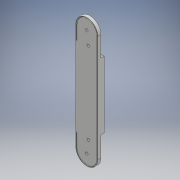
# Autodesk Inventor part: C-PAN-TOP
Saved by Autodesk Inventor 2018 (Build 220112000, 112)
## iProperties
Created: 2018-01-23
Part Number: C-PAN-TOP
Material: Generic
Document SubType Name: Modeling
Designer: gevon
Density: 1 g/cm^3
Appearance: Default
Author: gevon
Autodesk Inventor part; units mm, degrees
ref_plane "YZ Plane" through (0, 0, 0) normal (1, 0, 0) x (0, 1, 0)
ref_plane "XZ Plane" through (0, 0, 0) normal (0, 1, 0) x (-1, 0, 0)
ref_plane "XY Plane" through (0, 0, 0) normal (0, 0, 1) x (1, 0, 0)
sketch "Sketch1" plane through (0, 0, 0) normal (0, 1, 0) x (-1, 0, 0)
  arc A0 (17.5, 106.9997) -> (-17.5, 106.9997) centre (0, 106.9997) ccw
  arc A1 (-17.5, -63.0003) -> (17.5, -63.0003) centre (0, -63.0003) ccw
  line L0 (17.5, 106.9997) -> (17.5, -63.0003)
  line L1 (-17.5, 106.9997) -> (-17.5, -63.0003)
  circle A2 centre (0, 106.9997) radius 2
  circle A3 centre (0, -63.0003) radius 2
  point P0 (0, 0)
  dimension "d0" = 35
  dimension "d1" = 35
  dimension "d2" = 205
  dimension "d3" = 4
  dimension "d4" = 4
  constraints: 4 centre point, 4 end point, 4 point on circle, 2 coincident, 2 tangent, 2 vertical
  measures "d0" diameter of A0
  measures "d1" diameter of A1
  measures "d3" diameter of A2
  measures "d4" diameter of A3
extrude "Extrusion1" add sketch "Sketch1" along normal blind 5
sketch "Sketch2" plane through (0, 5, 0) normal (0, 1, 0) x (1, 0, 0)
  circle A0 centre (2.5, 43.0003) radius 2
  circle A1 centre (2.5, -86.9997) radius 2
  line L0 (-17.5, 63.0003) -> (-17.5, -106.9997) projected
  circle A2 centre (0, 63.0003) radius 2 projected
  circle A3 centre (0, -106.9997) radius 2 projected
  point P0 (0, 0)
  dimension "d7" = 4
  dimension "d8" = 4
  dimension "d9" = 20
  dimension "d10" = 20
  dimension "d11" = 20
  constraints: 2 centre point
  measures "d7" diameter of A0
  measures "d8" diameter of A1
  measures "d9" distance from line of L0 A0.centre
  measures "d10" vertical distance of A2.centre A0.centre
  measures "d11" vertical distance of A3.centre A1.centre
extrude "Extrusion2" cut sketch "Sketch2" against normal blind 5 contours A0 | A1
sketch "Sketch3" plane through (0, 5, 0) normal (0, 1, 0) x (1, 0, 0)
  line L0 (-17.5, 63.0003) -> (-17.5, -106.9997) projected
  line L1 (17.5, -106.9997) -> (17.5, 63.0003) projected
  line L2 (-17.5, 31.0003) -> (17.5, 31.0003)
  line L3 (17.5, 31.0003) -> (17.5, -74.9997)
  line L4 (17.5, -74.9997) -> (-17.5, -74.9997)
  line L5 (-17.5, -74.9997) -> (-17.5, 31.0003)
  circle A0 centre (2.5, 43.0003) radius 2 projected
  circle A1 centre (2.5, -86.9997) radius 2 projected
  point P0 (0, 0)
  dimension "d14" = 12
  dimension "d15" = 12
  constraints: 8 end point, 2 parallel, 2 point on line, 1 horizontal, 1 perpendicular
  measures "d14" distance from line of L2 A0.centre
  measures "d15" distance from line of L4 A1.centre
extrude "Extrusion3" add sketch "Sketch3" along normal blind 5 contours L2 L1 L4 L0
sketch "Sketch4" plane through (0, 10, 0) normal (0, 1, 0) x (1, 0, 0)
  point P0 (0, 0)
sketch "Sketch5" plane through (0, 10, 0) normal (0, 1, 0) x (1, 0, 0)
  line L0 (-10.4855, -70.1364) -> (34.9467, -70.1364) construction
  line L1 (34.9467, -70.1364) -> (34.9467, -84.8837) construction
  line L2 (34.9467, -84.8837) -> (-10.4855, -84.8837) construction
  line L3 (-10.4855, -84.8837) -> (-10.4855, -70.1364) construction
  spline S0 degree 2 poles (-8.9862, -73.3005) (-9.2826, -73.3005) (-9.784, -73.1004) (-9.9668, -72.9004) knots 0 0 0 1 2 2 2
  spline S1 degree 2 poles (-9.9668, -72.9004) (-10.1495, -72.7028) (-10.3496, -72.1099) (-10.3496, -71.7246) knots 0 0 0 1 2 2 2
  spline S2 degree 2 poles (-10.3496, -71.7246) (-10.3496, -71.3418) (-10.1545, -70.7737) (-9.9692, -70.5637) knots 0 0 0 1 2 2 2
  spline S3 degree 2 poles (-9.9692, -70.5637) (-9.7864, -70.3587) (-9.2875, -70.1438) (-8.9788, -70.1438) knots 0 0 0 1 2 2 2
  spline S4 degree 2 poles (-8.9788, -70.1438) (-8.8256, -70.1438) (-8.5564, -70.1883) (-8.4428, -70.2229) knots 0 0 0 1 2 2 2
  spline S5 degree 2 poles (-8.4428, -70.2229) (-8.344, -70.255) (-8.1389, -70.3464) (-8.0377, -70.4007) knots 0 0 0 1 2 2 2
  line L4 (-8.0377, -70.4007) -> (-8.0377, -70.8898)
  line L5 (-8.0377, -70.8898) -> (-8.0698, -70.8898)
  spline S6 degree 2 poles (-8.0698, -70.8898) (-8.1241, -70.8404) (-8.2921, -70.702) (-8.4131, -70.6353) knots 0 0 0 1 2 2 2
  spline S7 degree 2 poles (-8.4131, -70.6353) (-8.5292, -70.5711) (-8.8034, -70.4896) (-8.9812, -70.4896) knots 0 0 0 1 2 2 2
  spline S8 degree 2 poles (-8.9812, -70.4896) (-9.1764, -70.4896) (-9.5246, -70.6502) (-9.6555, -70.8033) knots 0 0 0 1 2 2 2
  spline S9 degree 2 poles (-9.6555, -70.8033) (-9.784, -70.9589) (-9.9272, -71.4307) (-9.9272, -71.7246) knots 0 0 0 1 2 2 2
  spline S10 degree 2 poles (-9.9272, -71.7246) (-9.9272, -72.0383) (-9.7766, -72.4903) (-9.6457, -72.6459) knots 0 0 0 1 2 2 2
  spline S11 degree 2 poles (-9.6457, -72.6459) (-9.5172, -72.7966) (-9.1739, -72.9498) (-8.9812, -72.9498) knots 0 0 0 1 2 2 2
  spline S12 degree 2 poles (-8.9812, -72.9498) (-8.8059, -72.9498) (-8.507, -72.8633) (-8.3909, -72.7991) knots 0 0 0 1 2 2 2
  spline S13 degree 2 poles (-8.3909, -72.7991) (-8.2797, -72.7349) (-8.1142, -72.6015) (-8.0673, -72.5546) knots 0 0 0 1 2 2 2
  line L6 (-8.0673, -72.5546) -> (-8.0377, -72.5546)
  line L7 (-8.0377, -72.5546) -> (-8.0377, -73.0387)
  spline S14 degree 2 poles (-8.0377, -73.0387) (-8.1389, -73.0856) (-8.3168, -73.1721) (-8.4428, -73.2116) knots 0 0 0 1 2 2 2
  spline S15 degree 2 poles (-8.4428, -73.2116) (-8.5761, -73.256) (-8.8034, -73.3005) (-8.9862, -73.3005) knots 0 0 0 1 2 2 2
  line L8 (-6.6298, -72.0976) -> (-7.7833, -72.0976)
  line L9 (-7.7833, -72.0976) -> (-7.7833, -71.7271)
  line L10 (-7.7833, -71.7271) -> (-6.6298, -71.7271)
  line L11 (-6.6298, -71.7271) -> (-6.6298, -72.0976)
  spline S16 degree 2 poles (-4.2116, -71.117) (-4.2116, -71.3146) (-4.3524, -71.6703) (-4.4784, -71.7938) knots 0 0 0 1 2 2 2
  spline S17 degree 2 poles (-4.4784, -71.7938) (-4.6365, -71.9494) (-5.0638, -72.1099) (-5.3898, -72.1099) knots 0 0 0 1 2 2 2
  line L12 (-5.3898, -72.1099) -> (-5.7332, -72.1099)
  line L13 (-5.7332, -72.1099) -> (-5.7332, -73.2462)
  line L14 (-5.7332, -73.2462) -> (-6.1382, -73.2462)
  line L15 (-6.1382, -73.2462) -> (-6.1382, -70.1982)
  line L16 (-6.1382, -70.1982) -> (-5.3725, -70.1982)
  spline S18 degree 2 poles (-5.3725, -70.1982) (-5.1008, -70.1982) (-4.7204, -70.2871) (-4.5747, -70.3883) knots 0 0 0 1 2 2 2
  spline S19 degree 2 poles (-4.5747, -70.3883) (-4.4043, -70.5044) (-4.2116, -70.8626) (-4.2116, -71.117) knots 0 0 0 1 2 2 2
  spline S20 degree 2 poles (-4.634, -71.1294) (-4.634, -70.9713) (-4.7427, -70.7391) (-4.8538, -70.665) knots 0 0 0 1 2 2 2
  spline S21 degree 2 poles (-4.8538, -70.665) (-4.9502, -70.6008) (-5.207, -70.5489) (-5.3972, -70.5489) knots 0 0 0 1 2 2 2
  line L17 (-5.3972, -70.5489) -> (-5.7332, -70.5489)
  line L18 (-5.7332, -70.5489) -> (-5.7332, -71.7641)
  line L19 (-5.7332, -71.7641) -> (-5.4565, -71.7641)
  spline S22 degree 2 poles (-5.4565, -71.7641) (-5.2095, -71.7641) (-4.9057, -71.6851) (-4.8069, -71.5814) knots 0 0 0 1 2 2 2
  spline S23 degree 2 poles (-4.8069, -71.5814) (-4.7155, -71.49) (-4.634, -71.2751) (-4.634, -71.1294) knots 0 0 0 1 2 2 2
  line L20 (-4.1548, -73.2462) -> (-3.1273, -70.1982)
  line L21 (-3.1273, -70.1982) -> (-2.6283, -70.1982)
  line L22 (-2.6283, -70.1982) -> (-1.6008, -73.2462)
  line L23 (-1.6008, -73.2462) -> (-2.0281, -73.2462)
  line L24 (-2.0281, -73.2462) -> (-2.3048, -72.394)
  line L25 (-2.3048, -72.394) -> (-3.4681, -72.394)
  line L26 (-3.4681, -72.394) -> (-3.7448, -73.2462)
  line L27 (-3.7448, -73.2462) -> (-4.1548, -73.2462)
  line L28 (-2.4159, -72.0482) -> (-2.8877, -70.6131)
  line L29 (-2.8877, -70.6131) -> (-3.357, -72.0482)
  line L30 (-3.357, -72.0482) -> (-2.4159, -72.0482)
  line L31 (0.8692, -73.2462) -> (0.4147, -73.2462)
  line L32 (0.4147, -73.2462) -> (-0.9339, -70.6181)
  line L33 (-0.9339, -70.6181) -> (-0.9339, -73.2462)
  line L34 (-0.9339, -73.2462) -> (-1.3118, -73.2462)
  line L35 (-1.3118, -73.2462) -> (-1.3118, -70.1982)
  line L36 (-1.3118, -70.1982) -> (-0.7363, -70.1982)
  line L37 (-0.7363, -70.1982) -> (0.4913, -72.6114)
  line L38 (0.4913, -72.6114) -> (0.4913, -70.1982)
  line L39 (0.4913, -70.1982) -> (0.8692, -70.1982)
  line L40 (0.8692, -70.1982) -> (0.8692, -73.2462)
  line L41 (4.4359, -73.2462) -> (2.949, -73.2462)
  line L42 (2.949, -73.2462) -> (2.949, -72.9349)
  line L43 (2.949, -72.9349) -> (3.5022, -72.9349)
  line L44 (3.5022, -72.9349) -> (3.5022, -70.8922)
  line L45 (3.5022, -70.8922) -> (2.949, -70.8922)
  line L46 (2.949, -70.8922) -> (2.949, -70.6131)
  spline S24 degree 2 poles (2.949, -70.6131) (3.2626, -70.6131) (3.5591, -70.4353) (3.5788, -70.1883) knots 0 0 0 1 2 2 2
  line L47 (3.5788, -70.1883) -> (3.895, -70.1883)
  line L48 (3.895, -70.1883) -> (3.895, -72.9349)
  line L49 (3.895, -72.9349) -> (4.4359, -72.9349)
  line L50 (4.4359, -72.9349) -> (4.4359, -73.2462)
  line L51 (6.7231, -73.2462) -> (5.2362, -73.2462)
  line L52 (5.2362, -73.2462) -> (5.2362, -72.9349)
  line L53 (5.2362, -72.9349) -> (5.7895, -72.9349)
  line L54 (5.7895, -72.9349) -> (5.7895, -70.8922)
  line L55 (5.7895, -70.8922) -> (5.2362, -70.8922)
  line L56 (5.2362, -70.8922) -> (5.2362, -70.6131)
  spline S25 degree 2 poles (5.2362, -70.6131) (5.5499, -70.6131) (5.8463, -70.4353) (5.866, -70.1883) knots 0 0 0 1 2 2 2
  line L57 (5.866, -70.1883) -> (6.1822, -70.1883)
  line L58 (6.1822, -70.1883) -> (6.1822, -72.9349)
  line L59 (6.1822, -72.9349) -> (6.7231, -72.9349)
  line L60 (6.7231, -72.9349) -> (6.7231, -73.2462)
  spline S26 degree 2 poles (9.1808, -71.7222) (9.1808, -72.5422) (8.7041, -73.3104) (8.2076, -73.3104) knots 0 0 0 1 2 2 2
  spline S27 degree 2 poles (8.2076, -73.3104) (7.7037, -73.3104) (7.232, -72.5274) (7.232, -71.7246) knots 0 0 0 1 2 2 2
  spline S28 degree 2 poles (7.232, -71.7246) (7.232, -70.8996) (7.7087, -70.1364) (8.2076, -70.1364) knots 0 0 0 1 2 2 2
  spline S29 degree 2 poles (8.2076, -70.1364) (8.709, -70.1364) (9.1808, -70.9268) (9.1808, -71.7222) knots 0 0 0 1 2 2 2
  spline S30 degree 2 poles (8.6572, -72.6509) (8.7164, -72.5002) (8.7658, -72.0358) (8.7658, -71.7222) knots 0 0 0 1 2 2 2
  spline S31 degree 2 poles (8.7658, -71.7222) (8.7658, -71.4085) (8.7164, -70.9466) (8.6547, -70.791) knots 0 0 0 1 2 2 2
  spline S32 degree 2 poles (8.6547, -70.791) (8.5929, -70.6353) (8.3781, -70.4748) (8.2076, -70.4748) knots 0 0 0 1 2 2 2
  spline S33 degree 2 poles (8.2076, -70.4748) (8.0372, -70.4748) (7.8174, -70.6353) (7.7531, -70.7959) knots 0 0 0 1 2 2 2
  spline S34 degree 2 poles (7.7531, -70.7959) (7.6914, -70.9515) (7.6469, -71.4258) (7.6469, -71.7246) knots 0 0 0 1 2 2 2
  spline S35 degree 2 poles (7.6469, -71.7246) (7.6469, -72.0457) (7.6864, -72.4755) (7.7507, -72.6435) knots 0 0 0 1 2 2 2
  spline S36 degree 2 poles (7.7507, -72.6435) (7.8099, -72.8016) (8.0298, -72.972) (8.2076, -72.972) knots 0 0 0 1 2 2 2
  spline S37 degree 2 poles (8.2076, -72.972) (8.3756, -72.972) (8.5954, -72.8114) (8.6572, -72.6509) knots 0 0 0 1 2 2 2
  spline S38 degree 2 poles (11.468, -71.7222) (11.468, -72.5422) (10.9913, -73.3104) (10.4949, -73.3104) knots 0 0 0 1 2 2 2
  spline S39 degree 2 poles (10.4949, -73.3104) (9.991, -73.3104) (9.5192, -72.5274) (9.5192, -71.7246) knots 0 0 0 1 2 2 2
  spline S40 degree 2 poles (9.5192, -71.7246) (9.5192, -70.8996) (9.9959, -70.1364) (10.4949, -70.1364) knots 0 0 0 1 2 2 2
  spline S41 degree 2 poles (10.4949, -70.1364) (10.9963, -70.1364) (11.468, -70.9268) (11.468, -71.7222) knots 0 0 0 1 2 2 2
  spline S42 degree 2 poles (10.9444, -72.6509) (11.0037, -72.5002) (11.0531, -72.0358) (11.0531, -71.7222) knots 0 0 0 1 2 2 2
  spline S43 degree 2 poles (11.0531, -71.7222) (11.0531, -71.4085) (11.0037, -70.9466) (10.9419, -70.791) knots 0 0 0 1 2 2 2
  spline S44 degree 2 poles (10.9419, -70.791) (10.8802, -70.6353) (10.6653, -70.4748) (10.4949, -70.4748) knots 0 0 0 1 2 2 2
  spline S45 degree 2 poles (10.4949, -70.4748) (10.3244, -70.4748) (10.1046, -70.6353) (10.0404, -70.7959) knots 0 0 0 1 2 2 2
  spline S46 degree 2 poles (10.0404, -70.7959) (9.9786, -70.9515) (9.9342, -71.4258) (9.9342, -71.7246) knots 0 0 0 1 2 2 2
  spline S47 degree 2 poles (9.9342, -71.7246) (9.9342, -72.0457) (9.9737, -72.4755) (10.0379, -72.6435) knots 0 0 0 1 2 2 2
  spline S48 degree 2 poles (10.0379, -72.6435) (10.0972, -72.8016) (10.317, -72.972) (10.4949, -72.972) knots 0 0 0 1 2 2 2
  spline S49 degree 2 poles (10.4949, -72.972) (10.6628, -72.972) (10.8826, -72.8114) (10.9444, -72.6509) knots 0 0 0 1 2 2 2
  spline S50 degree 2 poles (13.7553, -71.7222) (13.7553, -72.5422) (13.2786, -73.3104) (12.7821, -73.3104) knots 0 0 0 1 2 2 2
  spline S51 degree 2 poles (12.7821, -73.3104) (12.2782, -73.3104) (11.8064, -72.5274) (11.8064, -71.7246) knots 0 0 0 1 2 2 2
  spline S52 degree 2 poles (11.8064, -71.7246) (11.8064, -70.8996) (12.2831, -70.1364) (12.7821, -70.1364) knots 0 0 0 1 2 2 2
  spline S53 degree 2 poles (12.7821, -70.1364) (13.2835, -70.1364) (13.7553, -70.9268) (13.7553, -71.7222) knots 0 0 0 1 2 2 2
  spline S54 degree 2 poles (13.2316, -72.6509) (13.2909, -72.5002) (13.3403, -72.0358) (13.3403, -71.7222) knots 0 0 0 1 2 2 2
  spline S55 degree 2 poles (13.3403, -71.7222) (13.3403, -71.4085) (13.2909, -70.9466) (13.2292, -70.791) knots 0 0 0 1 2 2 2
  spline S56 degree 2 poles (13.2292, -70.791) (13.1674, -70.6353) (12.9525, -70.4748) (12.7821, -70.4748) knots 0 0 0 1 2 2 2
  spline S57 degree 2 poles (12.7821, -70.4748) (12.6117, -70.4748) (12.3918, -70.6353) (12.3276, -70.7959) knots 0 0 0 1 2 2 2
  spline S58 degree 2 poles (12.3276, -70.7959) (12.2659, -70.9515) (12.2214, -71.4258) (12.2214, -71.7246) knots 0 0 0 1 2 2 2
  spline S59 degree 2 poles (12.2214, -71.7246) (12.2214, -72.0457) (12.2609, -72.4755) (12.3251, -72.6435) knots 0 0 0 1 2 2 2
  spline S60 degree 2 poles (12.3251, -72.6435) (12.3844, -72.8016) (12.6042, -72.972) (12.7821, -72.972) knots 0 0 0 1 2 2 2
  spline S61 degree 2 poles (12.7821, -72.972) (12.9501, -72.972) (13.1699, -72.8114) (13.2316, -72.6509) knots 0 0 0 1 2 2 2
  line L61 (15.8721, -73.2462) -> (14.3851, -73.2462)
  line L62 (14.3851, -73.2462) -> (14.3851, -72.9349)
  line L63 (14.3851, -72.9349) -> (14.9384, -72.9349)
  line L64 (14.9384, -72.9349) -> (14.9384, -70.8922)
  line L65 (14.9384, -70.8922) -> (14.3851, -70.8922)
  line L66 (14.3851, -70.8922) -> (14.3851, -70.6131)
  spline S62 degree 2 poles (14.3851, -70.6131) (14.6988, -70.6131) (14.9952, -70.4353) (15.015, -70.1883) knots 0 0 0 1 2 2 2
  line L67 (15.015, -70.1883) -> (15.3311, -70.1883)
  line L68 (15.3311, -70.1883) -> (15.3311, -72.9349)
  line L69 (15.3311, -72.9349) -> (15.8721, -72.9349)
  line L70 (15.8721, -72.9349) -> (15.8721, -73.2462)
  point P0 (0, 0)
  constraints: 2 other
extrude "Extrusion4" cut sketch "Sketch5" against normal blind 1
sketch "Sketch6" plane through (0, 0, 0) normal (0, -1, 0) x (1, 0, 0)
  arc A0 (16.75, 106.9997) -> (-16.75, 106.9997) centre (0, 106.9997) ccw
  arc A1 (15.75, 106.9997) -> (-15.75, 106.9997) centre (0, 106.9997) ccw
  arc A2 (-16.75, -63.0003) -> (16.75, -63.0003) centre (0, -63.0003) ccw
  arc A3 (-15.75, -63.0003) -> (15.75, -63.0003) centre (0, -63.0003) ccw
  line L0 (16.75, 106.9997) -> (16.75, -63.0003)
  line L1 (15.75, -63.0003) -> (15.75, 106.9997)
  line L2 (-15.75, -63.0003) -> (-15.75, -41.7669)
  line L3 (-15.75, -41.7669) -> (-16.75, -41.7669)
  line L4 (-16.75, -41.7669) -> (-16.75, -63.0003)
  line L5 (-15.75, 106.9997) -> (-15.75, 84.8601)
  line L6 (-15.75, 84.8601) -> (-16.75, 84.8601)
  line L7 (-16.75, 84.8601) -> (-16.75, 106.9997)
  arc A4 (-17.5, -63.0003) -> (17.5, -63.0003) centre (0, -63.0003) ccw projected
  point P0 (0, 0)
  dimension "d20" = 33.5
  dimension "d21" = 31.5
  dimension "d22" = 33.5
  dimension "d23" = 31.5
  dimension "d24" = 0
  dimension "d25" = 0.75
  constraints: 16 end point, 8 point on circle, 4 centre point, 4 point on line, 3 perpendicular, 1 coincident, 1 tangent
  measures "d20" diameter of A0
  measures "d21" diameter of A1
  measures "d22" diameter of A2
  measures "d23" diameter of A3
  measures "d24" distance of A2.centre A4.centre
  measures "d25" radial gap between concentric circles of A4 A2
extrude "Extrusion5" cut sketch "Sketch6" against normal blind 2
body "Solid1"
